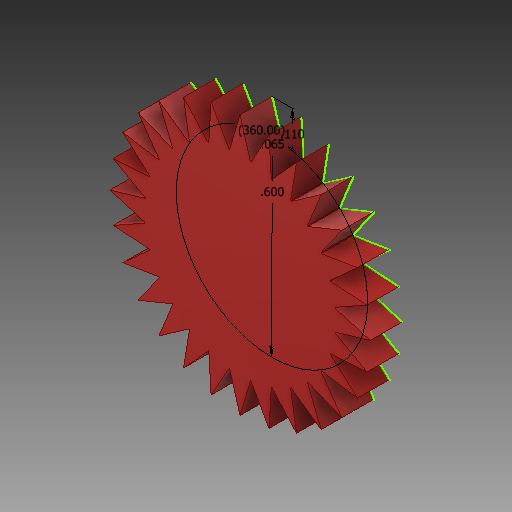
# Autodesk Inventor part: Big Gear Phone Case Mech
Saved by Autodesk Inventor 2018 (Build 220112000, 112)
## iProperties
Created: 2018-09-18
Part Number: Big Gear Phone Case Mech
Material: Generic
Document SubType Name: Modeling
Designer: User
Density: 1 g/cm^3
Appearance: Orange-Red
Author: User
Autodesk Inventor part; units mm, degrees
ref_plane "YZ Plane" through (0, 0, 0) normal (1, 0, 0) x (0, 1, 0)
ref_plane "XZ Plane" through (0, 0, 0) normal (0, 1, 0) x (-1, 0, 0)
ref_plane "XY Plane" through (0, 0, 0) normal (0, 0, 1) x (1, 0, 0)
sketch "Sketch3" plane through (0, 0, 0) normal (0, 0, 1) x (1, 0, 0)
  line L0 (-5.1387, 1.3261) -> (-4.3137, 4.1201)
  line L1 (-4.3137, 4.1201) -> (-3.4886, 1.3261)
  line L2 (-4.3137, 1.3261) -> (-5.1387, 1.3261) construction
  line L3 (-4.3137, 1.3261) -> (-4.3137, 1.6791) construction
  circle A0 centre (-4.3137, -6.2491) radius 7.62 construction
  circle A1 centre (-4.3137, -6.2491) radius 7.62 construction
  line L4 (-6.8037, 0.9526) -> (-6.621, 3.8601)
  line L5 (-6.621, 3.8601) -> (-5.1949, 1.3198)
  circle A2 centre (-4.3137, -6.2491) radius 7.62 construction
  line L6 (-8.3438, 0.218) -> (-8.8127, 3.0933)
  line L7 (-8.8127, 3.0933) -> (-6.8571, 0.9339)
  circle A3 centre (-4.3137, -6.2491) radius 7.62 construction
  line L8 (-9.6818, -0.841) -> (-10.7788, 1.8579)
  line L9 (-10.7788, 1.8579) -> (-8.3917, 0.1879)
  circle A4 centre (-4.3137, -6.2491) radius 7.62 construction
  line L10 (-10.7506, -2.1711) -> (-12.4206, 0.216)
  line L11 (-12.4206, 0.216) -> (-9.7218, -0.881)
  circle A5 centre (-4.3137, -6.2491) radius 7.62 construction
  line L12 (-11.4967, -3.7057) -> (-13.656, -1.75)
  line L13 (-13.656, -1.75) -> (-10.7807, -2.219)
  circle A6 centre (-4.3137, -6.2491) radius 7.62 construction
  line L14 (-11.8825, -5.3678) -> (-14.4229, -3.9417)
  line L15 (-14.4229, -3.9417) -> (-11.5154, -3.7591)
  circle A7 centre (-4.3137, -6.2491) radius 7.62 construction
  line L16 (-11.8889, -7.0741) -> (-14.6829, -6.2491)
  line L17 (-14.6829, -6.2491) -> (-11.8889, -5.424)
  circle A8 centre (-4.3137, -6.2491) radius 7.62 construction
  line L18 (-11.5154, -8.7391) -> (-14.4229, -8.5564)
  line L19 (-14.4229, -8.5564) -> (-11.8825, -7.1303)
  circle A9 centre (-4.3137, -6.2491) radius 7.62 construction
  line L20 (-10.7807, -10.2792) -> (-13.656, -10.7481)
  line L21 (-13.656, -10.7481) -> (-11.4967, -8.7925)
  circle A10 centre (-4.3137, -6.2491) radius 7.62 construction
  line L22 (-9.7218, -11.6172) -> (-12.4206, -12.7142)
  line L23 (-12.4206, -12.7142) -> (-10.7506, -10.3271)
  circle A11 centre (-4.3137, -6.2491) radius 7.62 construction
  line L24 (-8.3917, -12.686) -> (-10.7788, -14.356)
  line L25 (-10.7788, -14.356) -> (-9.6818, -11.6572)
  circle A12 centre (-4.3137, -6.2491) radius 7.62 construction
  line L26 (-6.8571, -13.4321) -> (-8.8127, -15.5914)
  line L27 (-8.8127, -15.5914) -> (-8.3438, -12.7161)
  circle A13 centre (-4.3137, -6.2491) radius 7.62 construction
  line L28 (-5.1949, -13.8179) -> (-6.621, -16.3583)
  line L29 (-6.621, -16.3583) -> (-6.8037, -13.4508)
  circle A14 centre (-4.3137, -6.2491) radius 7.62 construction
  line L30 (-3.4886, -13.8243) -> (-4.3137, -16.6183)
  line L31 (-4.3137, -16.6183) -> (-5.1387, -13.8243)
  circle A15 centre (-4.3137, -6.2491) radius 7.62 construction
  line L32 (-1.8237, -13.4508) -> (-2.0063, -16.3583)
  line L33 (-2.0063, -16.3583) -> (-3.4324, -13.8179)
  circle A16 centre (-4.3137, -6.2491) radius 7.62 construction
  line L34 (-0.2836, -12.7161) -> (0.1853, -15.5914)
  line L35 (0.1853, -15.5914) -> (-1.7703, -13.4321)
  circle A17 centre (-4.3137, -6.2491) radius 7.62 construction
  line L36 (1.0544, -11.6572) -> (2.1514, -14.356)
  line L37 (2.1514, -14.356) -> (-0.2357, -12.686)
  circle A18 centre (-4.3137, -6.2491) radius 7.62 construction
  line L38 (2.1233, -10.3271) -> (3.7933, -12.7142)
  line L39 (3.7933, -12.7142) -> (1.0944, -11.6172)
  circle A19 centre (-4.3137, -6.2491) radius 7.62 construction
  line L40 (2.8693, -8.7925) -> (5.0286, -10.7481)
  line L41 (5.0286, -10.7481) -> (2.1534, -10.2792)
  circle A20 centre (-4.3137, -6.2491) radius 7.62 construction
  line L42 (3.2552, -7.1303) -> (5.7955, -8.5564)
  line L43 (5.7955, -8.5564) -> (2.888, -8.7391)
  circle A21 centre (-4.3137, -6.2491) radius 7.62 construction
  line L44 (3.2615, -5.424) -> (6.0555, -6.2491)
  line L45 (6.0555, -6.2491) -> (3.2615, -7.0741)
  circle A22 centre (-4.3137, -6.2491) radius 7.62 construction
  line L46 (2.888, -3.7591) -> (5.7955, -3.9417)
  line L47 (5.7955, -3.9417) -> (3.2552, -5.3678)
  circle A23 centre (-4.3137, -6.2491) radius 7.62 construction
  line L48 (2.1534, -2.219) -> (5.0286, -1.75)
  line L49 (5.0286, -1.75) -> (2.8693, -3.7057)
  circle A24 centre (-4.3137, -6.2491) radius 7.62 construction
  line L50 (1.0944, -0.881) -> (3.7933, 0.216)
  line L51 (3.7933, 0.216) -> (2.1233, -2.1711)
  circle A25 centre (-4.3137, -6.2491) radius 7.62 construction
  line L52 (-0.2357, 0.1879) -> (2.1514, 1.8579)
  line L53 (2.1514, 1.8579) -> (1.0544, -0.841)
  circle A26 centre (-4.3137, -6.2491) radius 7.62 construction
  line L54 (-1.7703, 0.9339) -> (0.1853, 3.0933)
  line L55 (0.1853, 3.0933) -> (-0.2836, 0.218)
  circle A27 centre (-4.3137, -6.2491) radius 7.62 construction
  line L56 (-3.4324, 1.3198) -> (-2.0063, 3.8601)
  line L57 (-2.0063, 3.8601) -> (-1.8237, 0.9526)
  arc A28 (-10.7506, -2.1711) -> (-10.7807, -2.219) centre (-4.3137, -6.2491) ccw
  arc A29 (-11.4967, -3.7057) -> (-11.5154, -3.7591) centre (-4.3137, -6.2491) ccw
  arc A30 (-11.8825, -5.3678) -> (-11.8889, -5.424) centre (-4.3137, -6.2491) ccw
  arc A31 (-11.8889, -7.0741) -> (-11.8825, -7.1303) centre (-4.3137, -6.2491) ccw
  arc A32 (-11.5154, -8.7391) -> (-11.4967, -8.7925) centre (-4.3137, -6.2491) ccw
  arc A33 (-10.7807, -10.2792) -> (-10.7506, -10.3271) centre (-4.3137, -6.2491) ccw
  arc A34 (-9.7218, -11.6172) -> (-9.6818, -11.6572) centre (-4.3137, -6.2491) ccw
  arc A35 (-8.3917, -12.686) -> (-8.3438, -12.7161) centre (-4.3137, -6.2491) ccw
  arc A36 (-6.8571, -13.4321) -> (-6.8037, -13.4508) centre (-4.3137, -6.2491) ccw
  arc A37 (-5.1949, -13.8179) -> (-5.1387, -13.8243) centre (-4.3137, -6.2491) ccw
  arc A38 (-3.4886, -13.8243) -> (-3.4324, -13.8179) centre (-4.3137, -6.2491) ccw
  arc A39 (-1.8237, -13.4508) -> (-1.7703, -13.4321) centre (-4.3137, -6.2491) ccw
  arc A40 (-0.2836, -12.7161) -> (-0.2357, -12.686) centre (-4.3137, -6.2491) ccw
  arc A41 (1.0544, -11.6572) -> (1.0944, -11.6172) centre (-4.3137, -6.2491) ccw
  arc A42 (2.1233, -10.3271) -> (2.1534, -10.2792) centre (-4.3137, -6.2491) ccw
  arc A43 (2.8693, -8.7925) -> (2.888, -8.7391) centre (-4.3137, -6.2491) ccw
  arc A44 (3.2552, -7.1303) -> (3.2615, -7.0741) centre (-4.3137, -6.2491) ccw
  arc A45 (3.2615, -5.424) -> (3.2552, -5.3678) centre (-4.3137, -6.2491) ccw
  arc A46 (2.888, -3.7591) -> (2.8693, -3.7057) centre (-4.3137, -6.2491) ccw
  arc A47 (2.1534, -2.219) -> (2.1233, -2.1711) centre (-4.3137, -6.2491) ccw
  arc A48 (1.0944, -0.881) -> (1.0544, -0.841) centre (-4.3137, -6.2491) ccw
  arc A49 (-0.2357, 0.1879) -> (-0.2836, 0.218) centre (-4.3137, -6.2491) ccw
  arc A50 (-1.7703, 0.9339) -> (-1.8237, 0.9526) centre (-4.3137, -6.2491) ccw
  arc A51 (-3.4324, 1.3198) -> (-3.4886, 1.3261) centre (-4.3137, -6.2491) ccw
  arc A52 (-5.1387, 1.3261) -> (-5.1949, 1.3198) centre (-4.3137, -6.2491) ccw
  arc A53 (-6.8037, 0.9526) -> (-6.8571, 0.9339) centre (-4.3137, -6.2491) ccw
  arc A54 (-8.3438, 0.218) -> (-8.3917, 0.1879) centre (-4.3137, -6.2491) ccw
  arc A55 (-9.6818, -0.841) -> (-9.7218, -0.881) centre (-4.3137, -6.2491) ccw
  point P0 (0, 0)
  dimension "d21" = 1.6501
  dimension "d22" = 2.794
  dimension "d23" = 15.24
  dimension "d26" = 360
  constraints: 116 end point, 112 point on circle, 56 centre point, 3 coincident, 1 horizontal, 1 vertical, 196 other
  measures "d21" distance of L1.end L0.start
  measures "d22" distance from line of L2 L0.end
  measures "d23" diameter of A0
extrude "Extrusion3" add sketch "Sketch3" along normal blind 2.54
body "Solid2"
